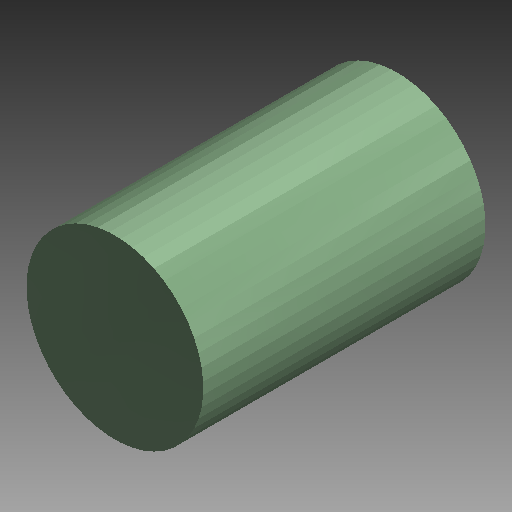
# Autodesk Inventor part: 100uF
Saved by Autodesk Inventor 2018.2 (Build 222227000, 227)
## iProperties
Part Number: 100uF
Material: Generic
Document SubType Name: Modeling
Designer: autocad
Appearance: C3,5-8, 100uF
Author: autocad
Autodesk Inventor part; units mm, degrees
ref_plane "YZ Plane" through (0, 0, 0) normal (1, 0, 0) x (0, 1, 0)
ref_plane "XZ Plane" through (0, 0, 0) normal (0, 1, 0) x (-1, 0, 0)
ref_plane "XY Plane" through (0, 0, 0) normal (0, 0, 1) x (1, 0, 0)
sketch "C3,5-8, 100uF_213" plane through (0, 0, 0) normal (0, 0, 1) x (1, 0, 0)
  line L0 (-3.994, 0.7945) -> (-3.8561, 1.309)
  line L1 (-3.8561, 1.309) -> (-3.6523, 1.8011)
  line L2 (-3.6523, 1.8011) -> (-3.3859, 2.2624)
  line L3 (-3.3859, 2.2624) -> (-3.0617, 2.685)
  line L4 (-3.0617, 2.685) -> (-2.685, 3.0617)
  line L5 (-2.685, 3.0617) -> (-2.2624, 3.3859)
  line L6 (-2.2624, 3.3859) -> (-1.8011, 3.6523)
  line L7 (-1.8011, 3.6523) -> (-1.309, 3.8561)
  line L8 (-1.309, 3.8561) -> (-0.7945, 3.994)
  line L9 (-0.7945, 3.994) -> (-0.2663, 4.0635)
  line L10 (-0.2663, 4.0635) -> (0, 4.0635)
  line L11 (0, 4.0635) -> (0.2663, 4.0635)
  line L12 (0.2663, 4.0635) -> (0.7944, 3.994)
  line L13 (0.7944, 3.994) -> (1.309, 3.8561)
  line L14 (1.309, 3.8561) -> (1.8011, 3.6523)
  line L15 (1.8011, 3.6523) -> (2.2624, 3.3859)
  line L16 (2.2624, 3.3859) -> (2.685, 3.0617)
  line L17 (2.685, 3.0617) -> (3.0616, 2.685)
  line L18 (3.0616, 2.685) -> (3.3859, 2.2624)
  line L19 (3.3859, 2.2624) -> (3.6522, 1.8011)
  line L20 (3.6522, 1.8011) -> (3.8561, 1.309)
  line L21 (3.8561, 1.309) -> (3.994, 0.7945)
  line L22 (3.994, 0.7945) -> (4.0635, 0.2663)
  line L23 (4.0635, 0.2663) -> (4.0635, -0.2663)
  line L24 (4.0635, -0.2663) -> (3.994, -0.7944)
  line L25 (3.994, -0.7944) -> (3.8561, -1.309)
  line L26 (3.8561, -1.309) -> (3.6522, -1.8011)
  line L27 (3.6522, -1.8011) -> (3.3859, -2.2624)
  line L28 (3.3859, -2.2624) -> (3.0616, -2.685)
  line L29 (3.0616, -2.685) -> (2.685, -3.0616)
  line L30 (2.685, -3.0616) -> (2.2624, -3.3859)
  line L31 (2.2624, -3.3859) -> (1.8011, -3.6522)
  line L32 (1.8011, -3.6522) -> (1.309, -3.8561)
  line L33 (1.309, -3.8561) -> (0.7944, -3.994)
  line L34 (0.7944, -3.994) -> (0.2663, -4.0635)
  line L35 (0.2663, -4.0635) -> (0, -4.0635)
  line L36 (0, -4.0635) -> (-0.2663, -4.0635)
  line L37 (-0.2663, -4.0635) -> (-0.7945, -3.994)
  line L38 (-0.7945, -3.994) -> (-1.309, -3.8561)
  line L39 (-1.309, -3.8561) -> (-1.8011, -3.6522)
  line L40 (-1.8011, -3.6522) -> (-2.2624, -3.3859)
  line L41 (-2.2624, -3.3859) -> (-2.685, -3.0616)
  line L42 (-2.685, -3.0616) -> (-3.0617, -2.685)
  line L43 (-3.0617, -2.685) -> (-3.3859, -2.2624)
  line L44 (-3.3859, -2.2624) -> (-3.6523, -1.8011)
  line L45 (-3.6523, -1.8011) -> (-3.8561, -1.309)
  line L46 (-3.8561, -1.309) -> (-3.994, -0.7944)
  line L47 (-3.994, -0.7944) -> (-4.0635, -0.2663)
  line L48 (-4.0635, -0.2663) -> (-4.0635, 0.2663)
  line L49 (-4.0635, 0.2663) -> (-3.994, 0.7945)
  constraints: 100 end point
extrude "Extrusion1" add sketch "C3,5-8, 100uF_213" along normal blind 13
body "Solid1"
